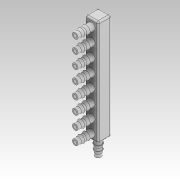
# Autodesk Inventor part: Manifold_8
Saved by Autodesk Inventor 2020 (Build 240168000, 168)
## iProperties
Created: 2020-08-02
Part Number: Manifold_8
Material: Generic
Document SubType Name: Modeling
Designer: DDeGo
Density: 1 g/cm^3
Appearance: Default
Author: DDeGo
Autodesk Inventor part; units mm, degrees
ref_plane "YZ Plane" through (0, 0, 0) normal (1, 0, 0) x (0, 1, 0)
ref_plane "XZ Plane" through (0, 0, 0) normal (0, 1, 0) x (-1, 0, 0)
sketch "Sketch1" plane through (0, 0, 0) normal (1, 0, 0) x (0, 1, 0)
  line L0 (1.75, 10) -> (1.05, 10)
  line L1 (0, 0) -> (0, 10) construction
  line L2 (0, 10) -> (1.05, 10) construction
  line L3 (1.8198, 8) -> (2.2759, 6.4097)
  line L4 (2.2759, 6.4097) -> (1.8759, 6.3957)
  line L5 (1.9282, 4.8957) -> (2.3843, 3.3053)
  line L6 (2.3843, 3.3053) -> (1.9843, 3.2914)
  line L7 (1.8759, 6.3957) -> (1.8198, 8) construction
  line L8 (1.8198, 8) -> (1.75, 10)
  line L9 (1.9282, 4.8957) -> (1.8759, 6.3957)
  line L10 (1.9843, 3.2914) -> (1.9282, 4.8957) construction
  line L11 (2.0992, 0) -> (1.9843, 3.2914)
  line L12 (1.05, 10) -> (1.05, 0)
  line L13 (1.05, 0) -> (2.0992, 0)
  line L14 (1.05, 0) -> (0, 0) construction
  dimension "d0" = 1.75
  dimension "d1" = 0.7
  dimension "d3" = 0.4
  dimension "d5" = 10
  dimension "d6" = 2
  dimension "d7" = 1.5
  dimension "d14" = 14
  dimension "d48" = 2
  constraints: 30 end point, 12 perpendicular, 2 horizontal, 2 parallel, 2 vertical
  measures "d0" distance of L1.end L0.start
  measures "d1" distance of L0.start L0.end
  measures "d3" horizontal distance of L3.end L4.end
  measures "d5" vertical distance of L11.start L0.start
  measures "d6" vertical distance of L0.end L3.start
  measures "d7" vertical distance of L4.end L5.start
  measures "d14" angle of L3 L7
  measures "d48" angle of L12 L8
revolve "Revolution1" add sketch "Sketch1" angle 360 about axis through (0, 0, 0) along (0, 0, 1)
pattern_linear "Rectangular Pattern1" count 8 spacing 8 along (0, 1, 0) of "Revolution1"
sketch "Sketch5" plane through (0, 0, 0) normal (0, 0, -1) x (-1, 0, 0)
  line L0 (4, 60) -> (-4, 60)
  line L1 (-4, 60) -> (-4, -4)
  line L2 (-4, -4) -> (4, -4)
  line L3 (4, -4) -> (4, 60)
  circle A0 centre (0, 56) radius 1.05 projected
  circle A1 centre (0, 48) radius 1.05 projected
  circle A2 centre (0, 40) radius 1.05 projected
  circle A3 centre (0, 32) radius 1.05 projected
  circle A4 centre (0, 24) radius 1.05 projected
  circle A5 centre (0, 16) radius 1.05 projected
  circle A6 centre (0, 8) radius 1.05 projected
  circle A7 centre (0, 0) radius 1.05 projected
  dimension "d50" = 4
  dimension "d51" = 4
  dimension "d55" = 4
  dimension "d56" = 4
  constraints: 8 end point, 2 parallel, 1 horizontal, 1 perpendicular
  measures "d50" distance from line of point (0, 0) L3
  measures "d51" distance from line of L1 point (0, 0)
  measures "d55" distance from line of L0 A0.centre
  measures "d56" distance from line of L2 point (0, 0)
extrude "Extrusion3" add sketch "Sketch5" along normal blind 8
ref_plane "Work Plane1" through (0, 0, -4) normal (0, 0, -1) x (-1, 0, 0)
sketch "Sketch6" plane through (-4, -4, 0) normal (0, -1, 0) x (1, 0, 0)
  line L0 (5.05, -8) -> (2.95, -8) construction
  circle A0 centre (4, -4) radius 1.75
  line L1 (9.6, -4) -> (-1.6, -4) construction
  line L2 (8, -8) -> (0, -8) projected
  line L3 (4, -8) -> (4, 0) construction
  dimension "d59" = 3.5
  constraints: 3 midpoint, 2 end point, 1 centre point, 1 coincident, 1 vertical
  measures "d59" diameter of A0
extrude "Extrusion4" cut sketch "Sketch6" against normal blind 61.2
sketch "Sketch7" plane through (0, 0, -8) normal (0, 0, -1) x (-1, 0, 0)
  circle A0 centre (0, 0) radius 1.05 projected
  line L0 (4, -4) -> (4, 60) projected
  line L1 (4, 60) -> (-4, 60) projected
  line L2 (-4, 60) -> (-4, -4) projected
  line L3 (-4, -4) -> (4, -4) projected
  circle A1 centre (0, 0) radius 1.05 projected
  circle A2 centre (0, 8) radius 1.05 projected
  circle A3 centre (0, 16) radius 1.05 projected
  circle A4 centre (0, 24) radius 1.05 projected
  circle A5 centre (0, 32) radius 1.05 projected
  circle A6 centre (0, 40) radius 1.05 projected
  circle A7 centre (0, 48) radius 1.05 projected
  circle A8 centre (0, 56) radius 1.05 projected
extrude "Extrusion5" add sketch "Sketch7" against normal up to surface contours A0 | A2 | A3 | A4 | A5 | A6 | A7 | A8 round surface about axis through (0, -4, -4) along (0, 1, 0) radius 1.75 far side no
sketch "Sketch8" plane through (0, 0, -4) normal (0, 0, -1) x (-1, 0, 0)
  line L0 (1.75, -4) -> (-1.75, -4) construction
  line L1 (1.9283, -8.8947) -> (1.8759, -10.3947)
  line L2 (2.2761, -10.4087) -> (1.8759, -10.3947)
  line L3 (1.8198, -12) -> (2.2761, -10.4087)
  line L4 (1.8759, -10.3947) -> (1.8198, -12) construction
  line L5 (1.8198, -12) -> (1.75, -14)
  line L6 (1.75, -14) -> (1.05, -14)
  line L7 (0, -14) -> (1.05, -14) construction
  line L8 (1.9843, -7.2894) -> (1.9283, -8.8947) construction
  line L9 (1.9283, -8.8947) -> (2.3846, -7.3034)
  line L10 (1.05, -14) -> (1.05, -7.9699)
  line L11 (0, -4) -> (0, -14) construction
  line L12 (2.3846, -7.3034) -> (1.9843, -7.2894)
  line L13 (1.05, -4) -> (0, -4) construction
  line L14 (1.05, -4) -> (1.75, -4) construction
  line L15 (2.0992, -4) -> (1.9843, -7.2894)
  line L16 (1.75, -4) -> (1.05, -7.9699)
  line L17 (1.05, -7.9699) -> (1.05, -4) construction
  line L18 (1.75, -4) -> (2.0992, -4)
  point P0 (0, 0)
  dimension "d73" = 1.75
  dimension "d74" = 2
  dimension "d75" = 2
  dimension "d76" = 0.4005
  dimension "d77" = 14
  dimension "d78" = 1.5
  dimension "d80" = 0.7
  dimension "d81" = 10
  dimension "d82" = 10
  constraints: 37 end point, 11 perpendicular, 4 collinear, 2 parallel, 1 midpoint, 1 point on line, 1 vertical
  measures "d73" distance from line of L5.end L11
  measures "d74" angle of L5 L10
  measures "d75" distance from line of L3.start L6
  measures "d76" distance of L2.start L1.end
  measures "d77" angle of L4 L3
  measures "d78" vertical distance of L9.start L1.end
  measures "d80" distance of L10.start L5.end
  measures "d81" distance between parallel lines of L14 L6
  measures "d82" angle of L10 L16
revolve "Revolution2" add sketch "Sketch8" angle 360 about axis through (0, -4, -4) along (0, -1, 0)
fillet "Fillet5" radius 1 1 edges at (2.0992, -4, -4)
fillet "Fillet6" radius 1 12 edges at (-4, 28, 0) (-4, 28, -8) (4, 28, 0) (0, -4, 0) (-4, -4, -4) (0, -4, -8) (4, -4, -4) (-4, 60, -4) (0, 60, 0) (0, 60, -8) (4, 28, -8) (4, 60, -4)
fillet "Fillet7" radius 2 8 edges at (1.05, 0.0028, -2.6) (1.05, 8.0028, -2.6) (1.05, 16.0028, -2.6) (1.05, 24.0028, -2.6) (1.05, 32.0028, -2.6) (1.05, 40.0028, -2.6) (1.05, 48.0028, -2.6) (1.05, 56.0028, -2.6)
body "Solid1"
